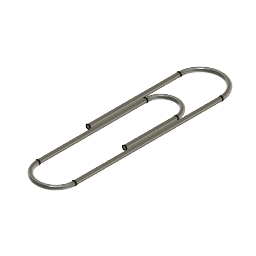
Paper clip (Autodesk Fusion 360 design; units mm, degrees)
part number: 2026-04-19-20-04-09-588
Autodesk Fusion 360 part; units mm, degrees
sketch "Sketch1" plane through (0, 0, 0) normal (0, 0, 1) x (1, 0, 0)
  line L0 (-20, 10) -> (-20, 26.25)
  line L1 (-20, 26.25) -> (-12.5, 26.25) construction
  line L2 (-12.5, 26.25) -> (-12.5, 0)
  line L3 (-12.5, 0) -> (-19, 0) construction
  line L4 (-19, 0) -> (-19, 19.25)
  line L5 (-19, 19.25) -> (-13.5, 19.25) construction
  line L6 (-13.5, 19.25) -> (-13.5, 10)
  arc A0 (-12.5, 26.25) -> (-20, 26.25) centre (-16.25, 26.25) ccw
  arc A1 (-19, 0) -> (-12.5, 0) centre (-15.75, 0) ccw
  arc A2 (-13.5, 19.25) -> (-19, 19.25) centre (-16.25, 19.25) ccw
  dimension "d1" = 16.25
  dimension "d2" = 7.5
  dimension "d3" = 26.25
  dimension "d4" = 6.5
  dimension "d5" = 19.25
  dimension "d6" = 5.5
  dimension "d7" = 9.25
  constraint vertical L0
  constraint perpendicular L0 L1
  constraint perpendicular L1 L2
  constraint perpendicular L2 L3
  constraint perpendicular L3 L4
  constraint perpendicular L4 L5
  constraint perpendicular L5 L6
  constraint tangent L0 A0
  constraint tangent L4 A1
  constraint tangent L4 A2
  measures "d1" distance of L0.start L0.end
  measures "d2" distance of L0.end L1.end
  measures "d3" distance of L1.end L2.end
  measures "d4" distance of L2.end L3.end
  measures "d5" distance of L3.end L4.end
  measures "d6" distance of L4.end L5.end
  measures "d7" distance of L5.end L6.end
sketch "Sketch2" plane through (0, 0, 0) normal (0, 1, 0) x (1, 0, 0)
  circle A0 centre (-20, 0) radius 0.375
  circle A1 through (-19.625, 0, 10) (-20.1875, 0.3248, 10) (-20.1875, -0.3248, 10)
  dimension "d8" = 0.75
  dimension "d9" = 0.75
  measures "d8" diameter of A0
sweep "Sweep1" add profiles "Sketch2" path "Sketch1" along L0 A0 L2 A1 L4 A2 L6 section 1 contours A1 in plane through (0, 10, 0) normal (0, 1, 0)
